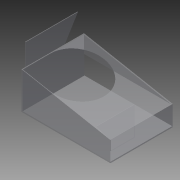
# Autodesk Inventor part: Hopper
Saved by Autodesk Inventor 2013 (Build 170138000, 138)
## iProperties
Created: 2013-03-22
Part Number: Hopper
Material: Polycarbonate, Clear
Document SubType Name: Modeling
Designer: actoennies
Mass: 1232.85 g
Surface Area: 8755.12 cm^2
Volume: 1379.02 cm^3
Density: 0.894 g/cm^3
Author: actoennies
Autodesk Inventor part; units mm, degrees
ref_plane "YZ Plane" through (0, 0, 0) normal (1, 0, 0) x (0, 1, 0)
ref_plane "XZ Plane" through (0, 0, 0) normal (0, 1, 0) x (-1, 0, 0)
ref_plane "XY Plane" through (0, 0, 0) normal (0, 0, 1) x (1, 0, 0)
sketch "Sketch1" plane through (0, 0, 0) normal (0, 0, 1) x (1, 0, 0)
  line L0 (0, 0) -> (0, 88.9)
  line L1 (0, 88.9) -> (467.8791, 0)
  line L2 (467.8791, 0) -> (0, 0)
  dimension "d0" = 88.9
  dimension "d4" = 476.25
  dimension "d5" = 90
  constraints: 6 end point, 1 vertical
  measures "d0" distance of L0.start L0.end
  measures "d4" distance of L0.end L1.end
  measures "d5" angle of L0 L2
extrude "Extrusion1" add sketch "Sketch1" along normal blind 3.175
sketch "Sketch2" plane through (0, 88.9, 0) normal (0.1866667, 0.9824233, 0) x (0.9824233, -0.1866667, 0)
  line L0 (0, 0) -> (476.25, 0) projected
  line L1 (0, 0) -> (0, -3.175) projected
  line L2 (476.25, -3.175) -> (0, -3.175) projected
  line L3 (476.25, 0) -> (476.25, -3.175) projected
  line L4 (0, -3.175) -> (0, -330.2)
  line L5 (0, -330.2) -> (476.25, -330.2)
  line L6 (476.25, -330.2) -> (476.25, -3.175)
  point P0 (16.5947, 0)
  dimension "d6" = 330.2
  constraints: 6 end point, 2 parallel, 1 perpendicular
  measures "d6" distance between parallel lines of L5 L0
extrude "Extrusion2" add sketch "Sketch2" along normal blind 3.175
sketch "Sketch3" plane through (0, 0, 0) normal (-1, 0, 0) x (0, 0, 1)
  line L0 (0, 0) -> (0, 88.9) projected
  line L1 (0, 0) -> (3.175, 0) projected
  line L2 (3.175, 88.9) -> (3.175, 0) projected
  line L3 (0, 88.9) -> (3.175, 88.9) projected
  line L4 (0, 88.9) -> (0, 92.075)
  line L5 (0, 92.075) -> (330.2, 92.075)
  line L6 (330.2, 92.075) -> (330.2, 0)
  line L7 (330.2, 0) -> (330.2, -101.6)
  line L8 (330.2, -101.6) -> (0, -101.6)
  line L9 (0, -101.6) -> (0, 0)
  dimension "d9" = 3.175
  dimension "d10" = 330.2
  dimension "d11" = 101.6
  constraints: 12 end point, 3 parallel, 3 perpendicular
  measures "d9" distance of L0.end L4.end
  measures "d10" distance of L4.end L5.end
  measures "d11" distance of L6.end L7.end
extrude "Extrusion3" add sketch "Sketch3" along normal blind 3.175
sketch "Sketch4" plane through (0, 0, 0) normal (0, 0, -1) x (-1, 0, 0)
  line L0 (0, 88.9) -> (-0.5927, 92.0192) projected
  line L1 (0, 92.075) -> (0, 88.9) projected
  line L2 (-0.5927, 92.0192) -> (0, 92.075)
  constraints: 2 end point
extrude "Extrusion4" add sketch "Sketch4" against normal blind 330.2
sketch "Sketch5" plane through (0, -101.6, 330.2) normal (0, 0, 1) x (1, 0, 0)
  line L0 (0, 190.5) -> (467.8791, 101.6) projected
  line L1 (467.8791, 101.6) -> (468.4718, 104.7192) projected
  line L2 (0.5927, 193.6192) -> (468.4718, 104.7192) projected
  line L3 (0.5927, 193.6192) -> (0, 193.675) projected
  line L4 (0, 193.675) -> (-3.175, 193.675) projected
  line L5 (-3.175, 0) -> (-3.175, 193.675) projected
  line L6 (0, 0) -> (-3.175, 0) projected
  line L7 (0, 0) -> (0, 190.5) projected
  line L8 (468.4718, 104.7192) -> (468.4718, 0)
  line L9 (468.4718, 0) -> (0, 0)
  point P0 (0, 101.6)
  constraints: 4 end point, 1 parallel, 1 perpendicular
extrude "Extrusion5" add sketch "Sketch5" along normal blind 3.175
sketch "Sketch6" plane through (0, -101.6, 330.2) normal (0, 0, -1) x (-1, 0, 0)
  line L0 (-467.8791, 101.6) -> (-468.4718, 104.7192) projected
  line L1 (-468.4718, 0) -> (-468.4718, 104.7192) projected
  line L2 (-467.8791, 101.6) -> (-468.4718, 101.6)
  point P0 (0, 101.6)
  constraints: 2 end point, 1 perpendicular, 1 point on line
extrude "Extrusion6" add sketch "Sketch6" along normal blind 330.2
sketch "Sketch7" plane through (468.4718, -101.6, 330.2) normal (1, 0, 0) x (0, 0, -1)
  line L0 (0, 0) -> (0, 101.6) projected
  line L1 (0, 101.6) -> (330.2, 101.6) projected
  line L2 (330.2, 104.7192) -> (330.2, 101.6) projected
  line L3 (-3.175, 104.7192) -> (330.2, 104.7192) projected
  line L4 (-3.175, 0) -> (-3.175, 104.7192) projected
  line L5 (0, 0) -> (-3.175, 0) projected
  line L6 (0, 0) -> (330.2, 0)
  line L7 (330.2, 0) -> (330.2, 101.6)
  constraints: 4 end point, 1 collinear, 1 perpendicular
extrude "Extrusion7" add sketch "Sketch7" along normal blind 3.175
sketch "Sketch8" plane through (0, -101.6, 0) normal (0, -1, 0) x (1, 0, 0)
  line L0 (0, 0) -> (0, 330.2) projected
  line L1 (471.6468, 333.375) -> (471.6468, 0) projected
  line L2 (-3.175, 333.375) -> (471.6468, 333.375) projected
  line L3 (-3.175, 0) -> (-3.175, 333.375) projected
  line L4 (0, 0) -> (-3.175, 0) projected
  line L5 (0, 0) -> (471.6468, 0)
  constraints: 2 end point, 1 collinear, 1 point on line
extrude "Extrusion8" add sketch "Sketch8" along normal blind 3.175
sketch "Sketch9" plane through (0, 88.9, 0) normal (-0.1866667, -0.9824233, 0) x (0.9824233, -0.1866667, 0)
  line L0 (0, 330.2) -> (476.25, 330.2) projected
  line L1 (0, 3.175) -> (0, 330.2) projected
  arc A0 (0, 184.15) -> (146.05, 330.2) centre (146.05, 184.15) ccw
  point P0 (16.5947, 0)
  dimension "d24" = 292.1
  constraints: 2 point on circle, 2 point on line, 2 tangent, 1 centre point
  measures "d24" diameter of A0
extrude "Extrusion9" cut sketch "Sketch9" against normal blind 3.175
sketch "Sketch10" plane through (471.6468, -101.6, 330.2) normal (1, 0, 0) x (0, 0, -1)
  line L0 (330.2, 104.7192) -> (-3.175, 104.7192) projected
  line L1 (-3.175, 104.7192) -> (-3.175, -3.175) projected
  line L2 (330.2, -3.175) -> (-3.175, -3.175) projected
  line L3 (123.825, 53.9192) -> (123.825, 206.3192)
  line L4 (123.825, 206.3192) -> (-79.375, 206.3192)
  line L5 (123.825, 53.9192) -> (-3.175, 53.9192)
  line L6 (-3.175, 53.9192) -> (-3.175, 104.7192)
  line L7 (-3.175, 104.7192) -> (-3.175, 104.7192)
  line L8 (-3.175, 104.7192) -> (-79.375, 206.3192)
  point P0 (330.2, 101.6)
  dimension "d30" = 152.4
  dimension "d31" = 203.2
  dimension "d32" = 127
  dimension "d33" = 50.8
  dimension "d34" = 0
  dimension "d35" = 0
  dimension "d47" = 0
  constraints: 12 end point, 3 perpendicular, 2 parallel
  measures "d30" distance of L3.start L3.end
  measures "d31" distance of L3.end L4.end
  measures "d32" distance of L3.start L5.end
  measures "d33" distance of L5.end L6.end
  measures "d34" distance of L6.end L7.end
  measures "d35" distance between parallel lines of L0 L7
  measures "d47" distance between parallel lines of L1 L6
extrude "Extrusion10" add sketch "Sketch10" along normal blind 3.175
sketch "Sketch11" plane through (-3.175, 0, 0) normal (-1, 0, 0) x (0, 0, 1)
  line L0 (333.375, 92.075) -> (333.375, -104.775) projected
  line L1 (0, 92.075) -> (333.375, 92.075) projected
  line L2 (311.15, 206.375) -> (31.75, 206.375)
  line L3 (311.15, 206.375) -> (311.15, 41.275)
  line L4 (311.15, 41.275) -> (101.6, 41.275)
  line L5 (101.6, 41.275) -> (101.6, 92.075)
  line L6 (101.6, 92.075) -> (31.75, 206.375)
  point P0 (0, 0)
  dimension "d39" = 279.4
  dimension "d40" = 165.1
  dimension "d41" = 209.55
  dimension "d42" = 50.8
  dimension "d43" = 0
  dimension "d44" = 22.225
  constraints: 10 end point, 2 parallel, 2 perpendicular
  measures "d39" distance of L2.start L2.end
  measures "d40" distance of L2.start L3.end
  measures "d41" distance of L3.end L4.end
  measures "d42" distance of L4.end L5.end
  measures "d43" distance from line of L1 L5.end
  measures "d44" distance between parallel lines of L0 L3
extrude "Extrusion11" add sketch "Sketch11" along normal blind 3.175
body "Solid1"
